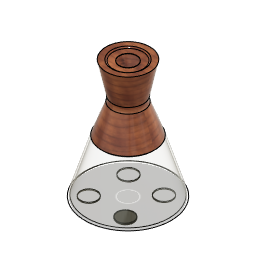
forme-maj-2023-12-19-c-ache v3 (Autodesk Fusion 360 design; units mm, degrees)
Autodesk Fusion 360 part; units mm, degrees
sketch "Esquisse1" plane through (0, 0, 0) normal (0, 0, 1) x (1, 0, 0)
  line L0 (0, 0) -> (-65, 0)
  line L1 (-65, 0) -> (-40, 80)
  line L2 (-40, 80) -> (0, 80)
  line L3 (0, 80) -> (0, 0)
  dimension "d1" = 65
  dimension "d2" = 40
  dimension "d3" = 80
  constraint coincident L0.start L3.end
  constraint horizontal L0
  constraint parallel L0 L2
  constraint perpendicular L0 L3
  measures "d1" distance of L0.start L0.end
  measures "d2" distance of L1.end L2.end
  measures "d3" vertical distance of L0.end L1.end
revolve "Révolution1" add sketch "Esquisse1" angle 360 about axis through (0, 80, 0) along (0, -1, 0) makes body 1
shell "Coque1" thickness 2 removed faces 1 at (0.2683, 80, 23.0112) on bodies 1
sketch "Esquisse2" plane through (0, 0, 0) normal (0, 0, 1) x (1, 0, 0)
  line L0 (0, 80) -> (-40, 80)
  line L1 (-40, 80) -> (-23.7921, 123.9523)
  line L2 (-23.1854, 132.2222) -> (-33, 179)
  line L3 (-33, 179) -> (0, 179)
  line L4 (0, 179) -> (0, 80)
  arc A0 (-23.7921, 123.9523) -> (-23.1854, 132.2222) centre (-37.8657, 129.1421) ccw
  point P0 (-22.2995, 128)
  dimension "d6" = 33
  dimension "d7" = 40
  dimension "d8" = 48
  dimension "d9" = 51
  dimension "d10" = 15
  constraint horizontal L0
  constraint horizontal L3
  constraint perpendicular L0 L4
  constraint coincident P0 L1
  constraint coincident P0 L2
  constraint tangent L1 A0
  constraint tangent L2 A0
  measures "d6" distance of L2.end L3.end
  measures "d7" distance of L0.start L0.end
  measures "d8" vertical distance of L0.end P0
  measures "d9" vertical distance of P0 L2.end
  measures "d10" radius of A0
revolve "Révolution2" add sketch "Esquisse2" angle 360 about axis through (0, 179, 0) along (0, -1, 0) separate body makes body 2
sketch "Esquisse3" plane through (0, 0, 0) normal (0, 0, 1) x (1, 0, 0)
  line L0 (-38, 80) -> (-38, 78)
  line L1 (-38, 78) -> (0, 78)
  line L2 (0, 78) -> (0, 80)
  line L3 (0, 80) -> (-38, 80)
  dimension "d12" = 2
  dimension "d13" = 38
  constraint vertical L0
  constraint perpendicular L0 L1
  constraint perpendicular L1 L2
  constraint perpendicular L0 L3
  measures "d12" distance of L0.start L0.end
  measures "d13" distance of L0.end L1.end
revolve "Révolution3" add sketch "Esquisse3" angle 360 about axis through (0, 1.75, 0) along (0, 1, 0) bodies 2
shell "Coque2" thickness 2 removed faces 1 at (-1.7057, 78, 19.7328) on bodies 2
hole "Perçage1" at (0, 179, 0) direction (0, -1, 0) diameter 26.5 depth 60 tip angle 180 counterbore diameter 45 counterbore depth 1.5 bodies 2
fillet "Congé1" radius 2.5 1 edges at (8.1363, 179, -20.9774) on bodies 2
hole "Perçage2" at (26.5907, 0, 30.5784) direction (0, 1, 0) diameter 25 depth 1.5 tip angle 180 bodies 1
hole "Perçage3" at (-26.5801, 0, -27.296) direction (0, 1, 0) diameter 25 depth 1.5 tip angle 180 bodies 1
hole "Perçage4" at (27.1994, 0, -27.296) direction (0, 1, 0) diameter 25 depth 1.5 tip angle 180 bodies 1
hole "Perçage6" at (-28.6252, 0, 30.7829) direction (0, 1, 0) diameter 25 depth 1.5 tip angle 180 bodies 1
sketch "Esquisse4" plane through (0, 0, 0) normal (0, 1, 0) x (1, 0, 0)
  circle A0 centre (0, 0) radius 12
  dimension "d38" = 24
  constraint coincident A0.centre origin
  measures "d38" diameter of A0
extrude "Extrusion1" add sketch "Esquisse4" along normal blind 2 separate body makes body 3
move_body "Déplacer1" bodies 3 to x (1, 0, 0) y (0, 1, 0) z (0, 0, 1) at (26.6, 0, 30.5)
move_body "Déplacer2" bodies 3 to x (1, 0, 0) y (0, 1, 0) z (0, 0, 1) at (0, -1, 0)
sketch "Esquisse5" plane through (0, 0, 0) normal (0, 1, 0) x (1, 0, 0)
  circle A0 centre (0, 0) radius 12
  dimension "d41" = 24
  constraint coincident A0.centre origin
  measures "d41" diameter of A0
equation "d13 = 40 mm - 2 mm"
named bodies: "Partie basse Pion résine", "Partie haute Pion bois", "Feutre anti derape"
